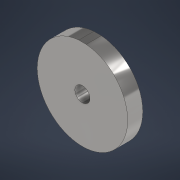
# Autodesk Inventor part: pinion
Saved by Autodesk Inventor 2021 (Build 250183000, 183)
## iProperties
Created: 2021-05-05
Part Number: pinion
Material: Steel, High Strength, Low Alloy
Document SubType Name: Modeling
Density: 7.85 g/cm^3
Appearance: Steel - Polished
Autodesk Inventor part; units mm, degrees
ref_plane "YZ Plane" through (0, 0, 0) normal (1, 0, 0) x (0, 1, 0)
ref_plane "XZ Plane" through (0, 0, 0) normal (0, 1, 0) x (-1, 0, 0)
ref_plane "XY Plane" through (0, 0, 0) normal (0, 0, 1) x (1, 0, 0)
sketch "Sketch1" plane through (0, 0, 0) normal (0, 0, 1) x (1, 0, 0)
  circle A0 centre (0, 0) radius 30
  dimension "d2" = 60
  constraints: 1 centre point, 1 coincident
  measures "d2" diameter of A0
extrude "Extrusion1" add sketch "Sketch1" along normal mid plane 10
sketch "Sketch2" plane through (0, 0, 0) normal (0, 0, 1) x (1, 0, 0)
  line L0 (2.5, 29.8957) -> (-2.5, 29.8957)
  circle A0 centre (0, 0) radius 30 projected
  line L1 (2.5, 30.9866) -> (-2.5, 30.9866)
  line L2 (-2.5, 30.9866) -> (-2.5, 29.8957)
  line L3 (2.5, 29.8957) -> (2.5, 30.9866)
  dimension "d3" = 5
  constraints: 8 end point, 2 horizontal, 2 point on circle, 1 parallel, 1 perpendicular
  measures "d3" distance of L0.start L0.end
extrude "Extrusion2" cut sketch "Sketch2" along normal mid plane 10 contours L0 A0 picked at (-0.2781, 29.9266)
sketch "Sketch3" plane through (0, 0, 5) normal (0, 0, 1) x (1, 0, 0)
  point P0 (0, 0)
  point P1 (0, 0)
  constraints: 1 coincident
hole "Hole1" at (0, 0, 5) direction (0, 0, -1) diameter 10 end through all
body "Solid1"
